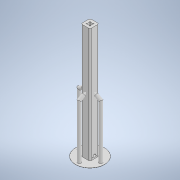
# Autodesk Inventor part: 130mm Rod Template
Saved by Autodesk Inventor 2022 (Build 260153000, 153)
## iProperties
Created: 2022-06-07
Part Number: 130mm Rod Template
Material: Generic
Document SubType Name: Modeling
Designer: Nick
Density: 1 g/cm^3
Appearance: Default
Author: Nick
Autodesk Inventor part; units mm, degrees
ref_plane "YZ Plane" through (0, 0, 0) normal (1, 0, 0) x (0, 1, 0)
ref_plane "XZ Plane" through (0, 0, 0) normal (0, 1, 0) x (-1, 0, 0)
ref_plane "XY Plane" through (0, 0, 0) normal (0, 0, 1) x (1, 0, 0)
sketch "Sketch1" plane through (0, 0, 0) normal (0, 1, 0) x (-1, 0, 0)
  circle A0 centre (0, 0) radius 2
  arc A1 (2.5, 2.179449) -> (2.5, -2.179449) centre (7, 0) ccw
  arc A2 (2.179449, -2.5) -> (-2.179449, -2.5) centre (0, -7) ccw
  arc A3 (-2.5, -2.179449) -> (-2.5, 2.179449) centre (-7, 0) ccw
  arc A4 (-2.179449, 2.5) -> (2.179449, 2.5) centre (0, 7) ccw
  line L0 (2.5, 2.5) -> (-2.5, 2.5)
  line L1 (-2.5, 2.5) -> (-2.5, -2.5)
  line L2 (-2.5, -2.5) -> (2.5, -2.5)
  line L3 (2.5, -2.5) -> (2.5, 2.5)
  line L4 (-5.5, -5.5) -> (-5.5, 5.5)
  line L5 (-5.5, 5.5) -> (5.5, 5.5)
  line L6 (5.5, 5.5) -> (5.5, -5.5)
  line L7 (5.5, -5.5) -> (-5.5, -5.5)
  point P0 (2.5, 0)
  point P1 (0, -2.5)
  dimension "d0" = 4
  dimension "d1" = 5
  dimension "d2" = 5
  dimension "d3" = 3
  constraints: 16 end point, 8 point on circle, 8 point on line, 5 centre point, 4 parallel, 4 tangent, 3 equal radius, 3 horizontal alignment, 3 perpendicular, 3 vertical alignment, 2 midpoint, 1 coincident, 1 horizontal, 3 other
  measures "d0" diameter of A0
  measures "d1" distance of L0.start L0.end
  measures "d2" radius of A4
  measures "d3" distance between parallel lines of L1 L4
extrude "Extrusion1" add sketch "Sketch1" along normal blind 137 contours A1 L3 | A4 L0 | A2 L2 | A3 L1 | L4 L5 L6 L7
sketch "Sketch2" plane through (5.5, 0, -5.5) normal (0, 0, -1) x (-1, 0, 0)
  line L0 (11, 137) -> (11, 0) construction
  line L1 (11, 0) -> (0, 0) construction
  line L2 (0, 0) -> (0, 137) construction
  line L3 (0, 137) -> (11, 137) construction
  line L4 (0, 0) -> (0, 137)
  line L5 (0, 137) -> (11, 137)
  line L6 (11, 0) -> (11, 137)
  line L7 (0, 0) -> (11, 0)
  line L8 (2.452472, 78.51013) -> (2.452472, 81.485981)
  line L9 (2.452472, 81.485981) -> (3.075324, 81.485981)
  line L10 (3.075324, 81.485981) -> (3.075324, 80.378688)
  line L11 (3.075324, 80.378688) -> (7.163412, 80.378688)
  line L12 (7.163412, 80.378688) -> (7.163412, 81.485981)
  line L13 (7.163412, 81.485981) -> (7.722002, 81.485981)
  spline S0 degree 2 poles (7.722002, 81.485981) (7.722002, 80.858185) (8.077917, 80.264993) (8.572245, 80.225446) knots 0 0 0 1 2 2 2
  line L14 (8.572245, 80.225446) -> (8.572245, 79.592707)
  line L15 (8.572245, 79.592707) -> (3.075324, 79.592707)
  line L16 (3.075324, 79.592707) -> (3.075324, 78.51013)
  line L17 (3.075324, 78.51013) -> (2.452472, 78.51013)
  line L18 (4.54842, 73.463047) -> (4.54842, 74.189709)
  line L19 (4.54842, 74.189709) -> (2.452472, 74.189709)
  line L20 (2.452472, 74.189709) -> (2.452472, 74.975689)
  line L21 (2.452472, 74.975689) -> (4.54842, 74.975689)
  line L22 (4.54842, 74.975689) -> (4.54842, 77.669774)
  line L23 (4.54842, 77.669774) -> (5.408549, 77.669774)
  line L24 (5.408549, 77.669774) -> (8.552472, 74.941086)
  line L25 (8.552472, 74.941086) -> (8.552472, 74.189709)
  line L26 (8.552472, 74.189709) -> (5.205875, 74.189709)
  line L27 (5.205875, 74.189709) -> (5.205875, 73.463047)
  line L28 (5.205875, 73.463047) -> (4.54842, 73.463047)
  line L29 (5.205875, 74.975689) -> (7.588533, 74.975689)
  line L30 (7.588533, 74.975689) -> (5.205875, 77.027148)
  line L31 (5.205875, 77.027148) -> (5.205875, 74.975689)
  spline S1 degree 2 poles (5.502472, 69.014101) (3.861305, 69.014101) (2.323946, 69.968153) (2.323946, 70.961751) knots 0 0 0 1 2 2 2
  spline S2 degree 2 poles (2.323946, 70.961751) (2.323946, 71.970179) (3.890964, 72.914344) (5.497528, 72.914344) knots 0 0 0 1 2 2 2
  spline S3 degree 2 poles (5.497528, 72.914344) (7.148582, 72.914344) (8.676054, 71.960292) (8.676054, 70.961751) knots 0 0 0 1 2 2 2
  spline S4 degree 2 poles (8.676054, 70.961751) (8.676054, 69.958266) (7.094206, 69.014101) (5.502472, 69.014101) knots 0 0 0 1 2 2 2
  spline S5 degree 2 poles (3.643801, 70.062075) (3.94534, 69.943436) (4.874676, 69.844571) (5.502472, 69.844571) knots 0 0 0 1 2 2 2
  spline S6 degree 2 poles (5.502472, 69.844571) (6.130267, 69.844571) (7.05466, 69.943436) (7.366086, 70.067018) knots 0 0 0 1 2 2 2
  spline S7 degree 2 poles (7.366086, 70.067018) (7.677512, 70.1906) (7.998825, 70.620665) (7.998825, 70.961751) knots 0 0 0 1 2 2 2
  spline S8 degree 2 poles (7.998825, 70.961751) (7.998825, 71.302837) (7.677512, 71.742788) (7.356199, 71.871313) knots 0 0 0 1 2 2 2
  spline S9 degree 2 poles (7.356199, 71.871313) (7.044773, 71.994895) (6.095665, 72.083874) (5.497528, 72.083874) knots 0 0 0 1 2 2 2
  spline S10 degree 2 poles (5.497528, 72.083874) (4.854903, 72.083874) (3.994773, 72.004782) (3.65863, 71.876257) knots 0 0 0 1 2 2 2
  spline S11 degree 2 poles (3.65863, 71.876257) (3.342261, 71.757618) (3.001175, 71.317667) (3.001175, 70.961751) knots 0 0 0 1 2 2 2
  spline S12 degree 2 poles (3.001175, 70.961751) (3.001175, 70.625608) (3.322488, 70.185657) (3.643801, 70.062075) knots 0 0 0 1 2 2 2
  line L32 (2.452472, 62.928931) -> (5.102066, 62.928931)
  spline S13 degree 2 poles (5.102066, 62.928931) (5.418436, 62.928931) (5.957253, 62.978363) (6.105551, 63.057456) knots 0 0 0 1 2 2 2
  spline S14 degree 2 poles (6.105551, 63.057456) (6.268679, 63.136548) (6.426864, 63.438088) (6.426864, 63.700081) knots 0 0 0 1 2 2 2
  spline S15 degree 2 poles (6.426864, 63.700081) (6.426864, 63.937358) (6.135211, 64.481119) (5.858387, 64.767828) knots 0 0 0 1 2 2 2
  spline S16 degree 2 poles (5.858387, 64.767828) (5.789182, 64.762885) (5.596394, 64.752999) (5.467869, 64.752999) knots 0 0 0 1 2 2 2
  line L33 (5.467869, 64.752999) -> (2.452472, 64.752999)
  line L34 (2.452472, 64.752999) -> (2.452472, 65.524149)
  line L35 (2.452472, 65.524149) -> (5.102066, 65.524149)
  spline S17 degree 2 poles (5.102066, 65.524149) (5.418436, 65.524149) (5.957253, 65.573582) (6.105551, 65.652675) knots 0 0 0 1 2 2 2
  spline S18 degree 2 poles (6.105551, 65.652675) (6.268679, 65.731767) (6.426864, 66.033307) (6.426864, 66.2953) knots 0 0 0 1 2 2 2
  spline S19 degree 2 poles (6.426864, 66.2953) (6.426864, 66.542464) (6.115438, 67.091167) (5.873217, 67.348218) knots 0 0 0 1 2 2 2
  line L36 (5.873217, 67.348218) -> (2.452472, 67.348218)
  line L37 (2.452472, 67.348218) -> (2.452472, 68.119368)
  line L38 (2.452472, 68.119368) -> (7.029943, 68.119368)
  line L39 (7.029943, 68.119368) -> (7.029943, 67.348218)
  line L40 (7.029943, 67.348218) -> (6.525729, 67.348218)
  spline S20 degree 2 poles (6.525729, 67.348218) (6.827269, 67.046678) (7.158468, 66.453485) (7.158468, 66.097569) knots 0 0 0 1 2 2 2
  spline S21 degree 2 poles (7.158468, 66.097569) (7.158468, 65.692221) (6.787723, 65.064425) (6.367545, 64.901297) knots 0 0 0 1 2 2 2
  spline S22 degree 2 poles (6.367545, 64.901297) (6.758063, 64.550324) (7.158468, 63.887926) (7.158468, 63.50235) knots 0 0 0 1 2 2 2
  spline S23 degree 2 poles (7.158468, 63.50235) (7.158468, 63.205754) (6.975567, 62.721313) (6.76795, 62.543355) knots 0 0 0 1 2 2 2
  spline S24 degree 2 poles (6.76795, 62.543355) (6.560332, 62.360454) (5.93748, 62.15778) (5.467869, 62.15778) knots 0 0 0 1 2 2 2
  line L41 (5.467869, 62.15778) -> (2.452472, 62.15778)
  line L42 (2.452472, 62.15778) -> (2.452472, 62.928931)
  line L43 (2.452472, 55.884765) -> (5.102066, 55.884765)
  spline S25 degree 2 poles (5.102066, 55.884765) (5.418436, 55.884765) (5.957253, 55.934198) (6.105551, 56.01329) knots 0 0 0 1 2 2 2
  spline S26 degree 2 poles (6.105551, 56.01329) (6.268679, 56.092383) (6.426864, 56.393922) (6.426864, 56.655916) knots 0 0 0 1 2 2 2
  spline S27 degree 2 poles (6.426864, 56.655916) (6.426864, 56.893193) (6.135211, 57.436953) (5.858387, 57.723663) knots 0 0 0 1 2 2 2
  spline S28 degree 2 poles (5.858387, 57.723663) (5.789182, 57.71872) (5.596394, 57.708833) (5.467869, 57.708833) knots 0 0 0 1 2 2 2
  line L44 (5.467869, 57.708833) -> (2.452472, 57.708833)
  line L45 (2.452472, 57.708833) -> (2.452472, 58.479984)
  line L46 (2.452472, 58.479984) -> (5.102066, 58.479984)
  spline S29 degree 2 poles (5.102066, 58.479984) (5.418436, 58.479984) (5.957253, 58.529417) (6.105551, 58.608509) knots 0 0 0 1 2 2 2
  spline S30 degree 2 poles (6.105551, 58.608509) (6.268679, 58.687601) (6.426864, 58.989141) (6.426864, 59.251135) knots 0 0 0 1 2 2 2
  spline S31 degree 2 poles (6.426864, 59.251135) (6.426864, 59.498298) (6.115438, 60.047002) (5.873217, 60.304052) knots 0 0 0 1 2 2 2
  line L47 (5.873217, 60.304052) -> (2.452472, 60.304052)
  line L48 (2.452472, 60.304052) -> (2.452472, 61.075203)
  line L49 (2.452472, 61.075203) -> (7.029943, 61.075203)
  line L50 (7.029943, 61.075203) -> (7.029943, 60.304052)
  line L51 (7.029943, 60.304052) -> (6.525729, 60.304052)
  spline S32 degree 2 poles (6.525729, 60.304052) (6.827269, 60.002512) (7.158468, 59.409319) (7.158468, 59.053404) knots 0 0 0 1 2 2 2
  spline S33 degree 2 poles (7.158468, 59.053404) (7.158468, 58.648055) (6.787723, 58.020259) (6.367545, 57.857131) knots 0 0 0 1 2 2 2
  spline S34 degree 2 poles (6.367545, 57.857131) (6.758063, 57.506159) (7.158468, 56.84376) (7.158468, 56.458185) knots 0 0 0 1 2 2 2
  spline S35 degree 2 poles (7.158468, 56.458185) (7.158468, 56.161588) (6.975567, 55.677148) (6.76795, 55.49919) knots 0 0 0 1 2 2 2
  spline S36 degree 2 poles (6.76795, 55.49919) (6.560332, 55.316289) (5.93748, 55.113614) (5.467869, 55.113614) knots 0 0 0 1 2 2 2
  line L52 (5.467869, 55.113614) -> (2.452472, 55.113614)
  line L53 (2.452472, 55.113614) -> (2.452472, 55.884765)
  point P0 (5.5, 0)
  dimension "d0" = 4
  dimension "d1" = 5
  dimension "d2" = 5
  dimension "d3" = 3
  constraints: 4 collinear, 1 vertical, 2 other
emboss "Emboss1" sketch "Sketch2" operation cut depth 0.2 direction (0, 0, 1) contours L8 L9 L10 L11 L12 L13 S0 L14 L15 L16 L17 | L18 L19 L20 L21 L22 L23 L24 L25 L26 L27 L28 | S1 S2 S3 S4 | L32 S13 S14 S15 S16 L33 L34 L35 S17 S18 S19 L36 L37 L38 L39 L40 S20 S21 S22 S23 S24 L41 L42 | L43 S25 S26 S27 S28 L44 L45 L46 S29 S30 S31 L47 L48 L49 L50 L51 S32 S33 S34 S35 S36 L52 L53
fillet "Fillet1" radius 2 4 edges at (-5.5, 68.5, 5.5) (-5.5, 68.5, -5.5) (5.5, 68.5, -5.5) (5.5, 68.5, 5.5)
sketch "Sketch3" plane through (0, 0, 0) normal (0, -1, 0) x (1, 0, 0)
  arc A0 (5.5, 3.5) -> (3.5, 5.5) centre (3.5, 3.5) ccw
  line L0 (-3.5, 5.5) -> (3.5, 5.5)
  arc A1 (-3.5, 5.5) -> (-5.5, 3.5) centre (-3.5, 3.5) ccw
  line L1 (-5.5, -3.5) -> (-5.5, 3.5)
  arc A2 (-5.5, -3.5) -> (-3.5, -5.5) centre (-3.5, -3.5) ccw
  line L2 (3.5, -5.5) -> (-3.5, -5.5)
  arc A3 (3.5, -5.5) -> (5.5, -3.5) centre (3.5, -3.5) ccw
  line L3 (5.5, 3.5) -> (5.5, -3.5)
  arc A4 (-2.5, -2.179449) -> (-2.5, 2.179449) centre (-7, 0) ccw
  line L4 (-2.5, 2.5) -> (-2.5, 2.179449)
  line L5 (-2.179449, 2.5) -> (-2.5, 2.5)
  arc A5 (-2.179449, 2.5) -> (2.179449, 2.5) centre (0, 7) ccw
  line L6 (2.5, 2.5) -> (2.179449, 2.5)
  line L7 (2.5, 2.179449) -> (2.5, 2.5)
  arc A6 (2.5, 2.179449) -> (2.5, -2.179449) centre (7, 0) ccw
  line L8 (2.5, -2.5) -> (2.5, -2.179449)
  line L9 (2.179449, -2.5) -> (2.5, -2.5)
  arc A7 (2.179449, -2.5) -> (-2.179449, -2.5) centre (0, -7) ccw
  line L10 (-2.5, -2.5) -> (-2.179449, -2.5)
  line L11 (-2.5, -2.179449) -> (-2.5, -2.5)
  point P0 (0, 0)
extrude "Extrusion2" add sketch "Sketch3" along normal blind 2 contours L3 A3 L2 A2 L1 A1 L0 A0 | A4 L4 L5 A5 L6 L7 A6 L8 L9 A7 L10 L11
sketch "Sketch4" plane through (5.5, 137, 3.5) normal (1, 0, 0) x (0, 0, -1)
  line L0 (5.679449, -137) -> (1.320551, -137)
  line L1 (6, -134) -> (1, -134)
  line L2 (1, -134) -> (1, -137)
  line L3 (1, -137) -> (6, -137)
  line L4 (6, -137) -> (6, -134)
  line L5 (6, -137) -> (4.267949, -134)
  line L6 (1, -137) -> (2.732051, -134)
  point P0 (3.5, -137)
  point P1 (1.320551, -137)
  dimension "d17" = 5
  dimension "d18" = 3
  dimension "d19" = 60
  dimension "d20" = 60
  constraints: 12 end point, 2 midpoint, 2 parallel, 2 point on line, 1 horizontal, 1 perpendicular
  measures "d17" distance of L3.end L2.end
  measures "d18" distance of L2.end L1.end
  measures "d19" angle of L3 L6
  measures "d20" angle of L3 L5
extrude "Extrusion3" cut sketch "Sketch4" against normal through all contours L0 L3 L6 L1 L5
sketch "Sketch5" plane through (0, -2, 0) normal (0, -1, 0) x (1, 0, 0)
  circle A0 centre (0, 0) radius 17.5
  dimension "d21" = 35
  constraints: 1 centre point, 1 coincident
  measures "d21" diameter of A0
extrude "Extrusion4" add sketch "Sketch5" against normal blind 0.2
sketch "Sketch6" plane through (0, -2, 0) normal (0, -1, 0) x (1, 0, 0)
  circle A0 centre (0, 0) radius 0.75
  dimension "d24" = 1.5
  constraints: 1 centre point, 1 coincident
  measures "d24" diameter of A0
extrude "Extrusion5" cut sketch "Sketch6" against normal through all
sketch "Sketch7" plane through (0, -1.8, 0) normal (0, 1, 0) x (1, 0, 0)
  circle A0 centre (13, 0) radius 2
  circle A1 centre (-13, 0) radius 2
  point P0 (0, 0)
  dimension "d27" = 13
  dimension "d28" = 13
  dimension "d29" = 4
  dimension "d30" = 4
  constraints: 2 centre point, 2 horizontal alignment
  measures "d27" distance of point (0, 0) A1.centre
  measures "d28" distance of A0.centre point (0, 0)
  measures "d29" diameter of A1
  measures "d30" diameter of A0
sketch "Sketch8" plane through (0, 0, 0) normal (0, 0, 1) x (1, 0, 0)
  line L0 (5.5, 137) -> (5.5, -1.8)
  line L1 (-5.5, 137) -> (-5.5, -1.8)
  line L2 (5.5, 137) -> (5.5, -1.8)
  line L3 (5.5, 67.6) -> (13, 60.1)
  line L4 (13, -1.8) -> (13, 60.1)
  line L5 (-5.5, 67.6) -> (-13, 63.269873)
  line L6 (-13, 63.269873) -> (-13, -1.8)
  line L7 (-5.5, 67.6) -> (-4.633975, 68.1)
  point P0 (0, 0)
  dimension "d31" = 135
  dimension "d32" = 120
  dimension "d38" = 1
  constraints: 10 end point, 2 midpoint, 2 vertical, 1 collinear
  measures "d31" angle of L4 L3
  measures "d32" angle of L6 L5
  measures "d38" distance of L5.start L7.end
sweep "Sweep1" add profiles "Sketch7" path "Sketch8" separate body path curves L6 L5 L7 contours A1
chamfer "Chamfer1" distance 2 angle 60 1 edges at (-5.634, 69.8321, 0) measured on face at (-5.384, 69.399, 0)
pattern_circular "Circular Pattern1" count 4 over 360 about axis through (0, -2, 0) along (0, 1, 0) of "Sweep1", "Chamfer1" bodies 2 skipped copies 4
body "Solid1"
body "Solid2"
